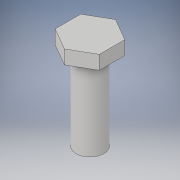
# Autodesk Inventor part: BM Beam Bolt
Saved by Autodesk Inventor 2017 (Build 210142000, 142)
## iProperties
Created: 2016-09-26
Part Number: BM Beam Bolt
Material: Generic
Document SubType Name: Modeling
Designer: Hanson
Density: 1 g/cm^3
Appearance: Default
Author: Hanson
Autodesk Inventor part; units mm, degrees
ref_plane "YZ Plane" through (0, 0, 0) normal (1, 0, 0) x (0, 1, 0)
ref_plane "XZ Plane" through (0, 0, 0) normal (0, 1, 0) x (-1, 0, 0)
ref_plane "XY Plane" through (0, 0, 0) normal (0, 0, 1) x (1, 0, 0)
sketch "Sketch1" plane through (0, 0, 0) normal (0, 1, 0) x (-1, 0, 0)
  circle A0 centre (0, 0) radius 3.175
  dimension "d0" = 6.35
  constraints: 1 centre point, 1 coincident
  measures "d0" diameter of A0
extrude "Extrusion1" add sketch "Sketch1" along normal blind 19.05
sketch "Sketch2" plane through (0, 19.05, 0) normal (0, 1, 0) x (1, 0, 0)
  line L0 (0, -5.8659) -> (-5.08, -2.9329)
  line L1 (-5.08, -2.9329) -> (-5.08, 2.9329)
  line L2 (-5.08, 2.9329) -> (0, 5.8659)
  line L3 (0, 5.8659) -> (5.08, 2.9329)
  line L4 (5.08, 2.9329) -> (5.08, -2.9329)
  line L5 (5.08, -2.9329) -> (0, -5.8659)
  point P0 (0, 0)
  point P1 (0, 0)
  dimension "d4" = 5.08
  constraints: 12 end point, 1 coincident, 13 other
  measures "d4" distance from line of L1 point (0, 0)
extrude "Extrusion2" add sketch "Sketch2" along normal blind 3.175
body "Solid1"
